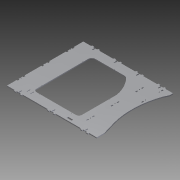
# Autodesk Inventor part: lateral esquerra
Saved by Autodesk Inventor 2012 SP1 (Build 160190100, 190)
## iProperties
Created: 2014-12-15
Part Number: lateral esquerra
Material: Default
Document SubType Name: Modeling
Designer: PRINCIPAL
Density: 1 g/cm^3
Author: PRINCIPAL
Autodesk Inventor part; units mm, degrees
ref_plane "YZ Plane" through (0, 0, 0) normal (1, 0, 0) x (0, 1, 0)
ref_plane "XZ Plane" through (0, 0, 0) normal (0, 1, 0) x (-1, 0, 0)
sketch "Boceto1" plane through (0, 0, 0) normal (0, 0, 1) x (1, 0, 0)
  line L0 (-98.625, -84.15) -> (-98.625, -94.05)
  line L1 (-98.625, -94.05) -> (-103.575, -94.05)
  line L2 (-103.575, -94.05) -> (-103.575, -84.15)
  line L3 (-103.575, -84.15) -> (-98.625, -84.15)
  line L4 (-98.625, -209.15) -> (-98.625, -219.05)
  line L5 (-98.625, -219.05) -> (-103.575, -219.05)
  line L6 (-103.575, -219.05) -> (-103.575, -209.15)
  line L7 (-103.575, -209.15) -> (-98.625, -209.15)
  line L8 (-98.625, -334.15) -> (-98.625, -344.05)
  line L9 (-98.625, -344.05) -> (-103.575, -344.05)
  line L10 (-103.575, -344.05) -> (-103.575, -334.15)
  line L11 (-103.575, -334.15) -> (-98.625, -334.15)
  line L12 (-98.625, -304.15) -> (-98.625, -314.05)
  line L13 (-98.625, -314.05) -> (-103.575, -314.05)
  line L14 (-103.575, -314.05) -> (-103.575, -304.15)
  line L15 (-103.575, -304.15) -> (-98.625, -304.15)
  line L16 (-98.625, -179.15) -> (-98.625, -189.05)
  line L17 (-98.625, -189.05) -> (-103.575, -189.05)
  line L18 (-103.575, -189.05) -> (-103.575, -179.15)
  line L19 (-103.575, -179.15) -> (-98.625, -179.15)
  line L20 (-98.625, -54.15) -> (-98.625, -64.05)
  line L21 (-98.625, -64.05) -> (-103.575, -64.05)
  line L22 (-103.575, -64.05) -> (-103.575, -54.15)
  line L23 (-103.575, -54.15) -> (-98.625, -54.15)
  arc A0 (-453.6069, -72.1) -> (-455.6069, -74.1) centre (-453.6069, -74.1) ccw
  arc A1 (-455.6069, -74.1) -> (-453.6069, -76.1) centre (-453.6069, -74.1) ccw
  arc A2 (-453.6069, -76.1) -> (-451.6069, -74.1) centre (-453.6069, -74.1) ccw
  arc A3 (-451.6069, -74.1) -> (-453.6069, -72.1) centre (-453.6069, -74.1) ccw
  arc A4 (-453.6069, -322.0506) -> (-455.6069, -324.0506) centre (-453.6069, -324.0506) ccw
  arc A5 (-455.6069, -324.0506) -> (-451.6069, -324.0506) centre (-453.6069, -324.051) ccw
  arc A6 (-451.6069, -324.0506) -> (-451.6069, -324.0506) centre (-453.6069, -324.0506) ccw
  arc A7 (-451.6069, -324.0506) -> (-453.6069, -322.0506) centre (-453.6069, -324.0506) ccw
  arc A8 (-453.6069, -197.1) -> (-455.6069, -199.1) centre (-453.6069, -199.1) ccw
  arc A9 (-455.6069, -199.1) -> (-453.6069, -201.1) centre (-453.6069, -199.1) ccw
  arc A10 (-453.6069, -201.1) -> (-451.6069, -199.1) centre (-453.6069, -199.1) ccw
  arc A11 (-451.6069, -199.1) -> (-453.6069, -197.1) centre (-453.6069, -199.1) ccw
  arc A12 (-101.1, -197.1) -> (-103.1, -199.1) centre (-101.1, -199.1) ccw
  arc A13 (-103.1, -199.1) -> (-101.1, -201.1) centre (-101.1, -199.1) ccw
  arc A14 (-101.1, -201.1) -> (-99.1, -199.1) centre (-101.1, -199.1) ccw
  arc A15 (-99.1, -199.1) -> (-101.1, -197.1) centre (-101.1, -199.1) ccw
  arc A16 (-101.1, -322.1) -> (-103.1, -324.1) centre (-101.1, -324.1) ccw
  arc A17 (-103.1, -324.1) -> (-101.1, -326.1) centre (-101.1, -324.1) ccw
  arc A18 (-101.1, -326.1) -> (-99.1, -324.1) centre (-101.1, -324.1) ccw
  arc A19 (-99.1, -324.1) -> (-101.1, -322.1) centre (-101.1, -324.1) ccw
  arc A20 (-101.1, -72.1) -> (-103.1, -74.1) centre (-101.1, -74.1) ccw
  arc A21 (-103.1, -74.1) -> (-101.1, -76.1) centre (-101.1, -74.1) ccw
  arc A22 (-101.1, -76.1) -> (-99.1, -74.1) centre (-101.1, -74.1) ccw
  arc A23 (-99.1, -74.1) -> (-101.1, -72.1) centre (-101.1, -74.1) ccw
  line L24 (-380.769, -353.9818) -> (-380.769, -368.4554)
  line L25 (-380.769, -368.4554) -> (-380.7613, -368.586)
  line L26 (-380.7613, -368.586) -> (-380.7385, -368.7128)
  line L27 (-380.7385, -368.7128) -> (-380.7016, -368.8352)
  line L28 (-380.7016, -368.8352) -> (-380.6511, -368.9525)
  line L29 (-380.6511, -368.9525) -> (-380.588, -369.0641)
  line L30 (-380.588, -369.0641) -> (-380.5128, -369.1694)
  line L31 (-380.5128, -369.1694) -> (-380.4265, -369.2678)
  line L32 (-380.4265, -369.2678) -> (-380.3297, -369.3584)
  line L33 (-380.3297, -369.3584) -> (-380.2231, -369.4409)
  line L34 (-380.2231, -369.4409) -> (-380.1077, -369.5144)
  line L35 (-380.1077, -369.5144) -> (-379.984, -369.5784)
  line L36 (-379.984, -369.5784) -> (-379.8529, -369.6321)
  line L37 (-379.8529, -369.6321) -> (-379.7151, -369.6751)
  line L38 (-379.7151, -369.6751) -> (-379.5713, -369.7065)
  line L39 (-379.5713, -369.7065) -> (-379.4224, -369.7259)
  line L40 (-379.4224, -369.7259) -> (-379.269, -369.7325)
  line L41 (-379.269, -369.7325) -> (-379.169, -369.7325)
  line L42 (-379.169, -369.7325) -> (-379.0156, -369.7259)
  line L43 (-379.0156, -369.7259) -> (-378.8667, -369.7065)
  line L44 (-378.8667, -369.7065) -> (-378.723, -369.6751)
  line L45 (-378.723, -369.6751) -> (-378.5851, -369.6321)
  line L46 (-378.5851, -369.6321) -> (-378.454, -369.5784)
  line L47 (-378.454, -369.5784) -> (-378.3303, -369.5144)
  line L48 (-378.3303, -369.5144) -> (-378.2149, -369.4409)
  line L49 (-378.2149, -369.4409) -> (-378.1083, -369.3584)
  line L50 (-378.1083, -369.3584) -> (-378.0115, -369.2678)
  line L51 (-378.0115, -369.2678) -> (-377.9252, -369.1694)
  line L52 (-377.9252, -369.1694) -> (-377.85, -369.0641)
  line L53 (-377.85, -369.0641) -> (-377.7869, -368.9525)
  line L54 (-377.7869, -368.9525) -> (-377.7364, -368.8352)
  line L55 (-377.7364, -368.8352) -> (-377.6995, -368.7128)
  line L56 (-377.6995, -368.7128) -> (-377.6768, -368.586)
  line L57 (-377.6768, -368.586) -> (-377.669, -368.4554)
  line L58 (-377.669, -368.4554) -> (-377.669, -353.9818)
  line L59 (-377.669, -353.9818) -> (-377.6768, -353.8512)
  line L60 (-377.6768, -353.8512) -> (-377.6995, -353.7244)
  line L61 (-377.6995, -353.7244) -> (-377.7364, -353.602)
  line L62 (-377.7364, -353.602) -> (-377.7869, -353.4847)
  line L63 (-377.7869, -353.4847) -> (-377.85, -353.373)
  line L64 (-377.85, -353.373) -> (-377.9252, -353.2677)
  line L65 (-377.9252, -353.2677) -> (-378.0115, -353.1694)
  line L66 (-378.0115, -353.1694) -> (-378.1083, -353.0787)
  line L67 (-378.1083, -353.0787) -> (-378.2149, -352.9963)
  line L68 (-378.2149, -352.9963) -> (-378.3303, -352.9228)
  line L69 (-378.3303, -352.9228) -> (-378.454, -352.8588)
  line L70 (-378.454, -352.8588) -> (-378.5851, -352.805)
  line L71 (-378.5851, -352.805) -> (-378.723, -352.7621)
  line L72 (-378.723, -352.7621) -> (-378.8667, -352.7306)
  line L73 (-378.8667, -352.7306) -> (-379.0156, -352.7113)
  line L74 (-379.0156, -352.7113) -> (-379.169, -352.7047)
  line L75 (-379.169, -352.7047) -> (-379.269, -352.7047)
  line L76 (-379.269, -352.7047) -> (-379.4224, -352.7113)
  line L77 (-379.4224, -352.7113) -> (-379.5713, -352.7306)
  line L78 (-379.5713, -352.7306) -> (-379.7151, -352.7621)
  line L79 (-379.7151, -352.7621) -> (-379.8529, -352.805)
  line L80 (-379.8529, -352.805) -> (-379.984, -352.8588)
  line L81 (-379.984, -352.8588) -> (-380.1077, -352.9228)
  line L82 (-380.1077, -352.9228) -> (-380.2231, -352.9963)
  line L83 (-380.2231, -352.9963) -> (-380.3297, -353.0787)
  line L84 (-380.3297, -353.0787) -> (-380.4265, -353.1694)
  line L85 (-380.4265, -353.1694) -> (-380.5128, -353.2677)
  line L86 (-380.5128, -353.2677) -> (-380.588, -353.373)
  line L87 (-380.588, -353.373) -> (-380.6511, -353.4847)
  line L88 (-380.6511, -353.4847) -> (-380.7016, -353.602)
  line L89 (-380.7016, -353.602) -> (-380.7385, -353.7244)
  line L90 (-380.7385, -353.7244) -> (-380.7613, -353.8512)
  line L91 (-380.7613, -353.8512) -> (-380.769, -353.9818)
  line L92 (-151.6064, -347.1) -> (-352.0892, -347.1)
  arc A24 (-367.0892, -332.1) -> (-352.0892, -347.1) centre (-352.0892, -332.1) ccw
  line L93 (-367.0892, -332.1) -> (-367.0892, -71.1)
  arc A25 (-347.0892, -51.1) -> (-367.0892, -71.1) centre (-347.0892, -71.1) ccw
  line L94 (-347.0892, -51.1) -> (-200.6138, -51.1)
  arc A26 (-186.1017, -57.3377) -> (-200.6138, -51.1) centre (-200.6138, -71.1) ccw
  arc A27 (-136.6064, -154.1) -> (-186.1017, -57.3377) centre (-325.8382, -189.8548) ccw
  line L95 (-136.6064, -154.1) -> (-136.6064, -332.1)
  arc A28 (-151.6064, -347.1) -> (-136.6064, -332.1) centre (-151.6064, -332.1) ccw
  line L96 (-361.769, -353.9818) -> (-361.769, -368.4554)
  line L97 (-361.769, -368.4554) -> (-361.7613, -368.586)
  line L98 (-361.7613, -368.586) -> (-361.7385, -368.7128)
  line L99 (-361.7385, -368.7128) -> (-361.7016, -368.8352)
  line L100 (-361.7016, -368.8352) -> (-361.6511, -368.9525)
  line L101 (-361.6511, -368.9525) -> (-361.588, -369.0641)
  line L102 (-361.588, -369.0641) -> (-361.5128, -369.1694)
  line L103 (-361.5128, -369.1694) -> (-361.4265, -369.2678)
  line L104 (-361.4265, -369.2678) -> (-361.3297, -369.3584)
  line L105 (-361.3297, -369.3584) -> (-361.2231, -369.4409)
  line L106 (-361.2231, -369.4409) -> (-361.1077, -369.5144)
  line L107 (-361.1077, -369.5144) -> (-360.984, -369.5784)
  line L108 (-360.984, -369.5784) -> (-360.8529, -369.6321)
  line L109 (-360.8529, -369.6321) -> (-360.7151, -369.6751)
  line L110 (-360.7151, -369.6751) -> (-360.5713, -369.7065)
  line L111 (-360.5713, -369.7065) -> (-360.4224, -369.7259)
  line L112 (-360.4224, -369.7259) -> (-360.269, -369.7325)
  line L113 (-360.269, -369.7325) -> (-360.169, -369.7325)
  line L114 (-360.169, -369.7325) -> (-360.0156, -369.7259)
  line L115 (-360.0156, -369.7259) -> (-359.8667, -369.7065)
  line L116 (-359.8667, -369.7065) -> (-359.723, -369.6751)
  line L117 (-359.723, -369.6751) -> (-359.5851, -369.6321)
  line L118 (-359.5851, -369.6321) -> (-359.454, -369.5784)
  line L119 (-359.454, -369.5784) -> (-359.3303, -369.5144)
  line L120 (-359.3303, -369.5144) -> (-359.2149, -369.4409)
  line L121 (-359.2149, -369.4409) -> (-359.1083, -369.3584)
  line L122 (-359.1083, -369.3584) -> (-359.0115, -369.2678)
  line L123 (-359.0115, -369.2678) -> (-358.9252, -369.1694)
  line L124 (-358.9252, -369.1694) -> (-358.85, -369.0641)
  line L125 (-358.85, -369.0641) -> (-358.7869, -368.9525)
  line L126 (-358.7869, -368.9525) -> (-358.7364, -368.8352)
  line L127 (-358.7364, -368.8352) -> (-358.6995, -368.7128)
  line L128 (-358.6995, -368.7128) -> (-358.6768, -368.586)
  line L129 (-358.6768, -368.586) -> (-358.669, -368.4554)
  line L130 (-358.669, -368.4554) -> (-358.669, -353.9818)
  line L131 (-358.669, -353.9818) -> (-358.6768, -353.8512)
  line L132 (-358.6768, -353.8512) -> (-358.6995, -353.7244)
  line L133 (-358.6995, -353.7244) -> (-358.7364, -353.602)
  line L134 (-358.7364, -353.602) -> (-358.7869, -353.4847)
  line L135 (-358.7869, -353.4847) -> (-358.85, -353.373)
  line L136 (-358.85, -353.373) -> (-358.9252, -353.2677)
  line L137 (-358.9252, -353.2677) -> (-359.0115, -353.1694)
  line L138 (-359.0115, -353.1694) -> (-359.1083, -353.0787)
  line L139 (-359.1083, -353.0787) -> (-359.2149, -352.9963)
  line L140 (-359.2149, -352.9963) -> (-359.3303, -352.9228)
  line L141 (-359.3303, -352.9228) -> (-359.454, -352.8588)
  line L142 (-359.454, -352.8588) -> (-359.5851, -352.805)
  line L143 (-359.5851, -352.805) -> (-359.723, -352.7621)
  line L144 (-359.723, -352.7621) -> (-359.8667, -352.7306)
  line L145 (-359.8667, -352.7306) -> (-360.0156, -352.7113)
  line L146 (-360.0156, -352.7113) -> (-360.169, -352.7047)
  line L147 (-360.169, -352.7047) -> (-360.269, -352.7047)
  line L148 (-360.269, -352.7047) -> (-360.4224, -352.7113)
  line L149 (-360.4224, -352.7113) -> (-360.5713, -352.7306)
  line L150 (-360.5713, -352.7306) -> (-360.7151, -352.7621)
  line L151 (-360.7151, -352.7621) -> (-360.8529, -352.805)
  line L152 (-360.8529, -352.805) -> (-360.984, -352.8588)
  line L153 (-360.984, -352.8588) -> (-361.1077, -352.9228)
  line L154 (-361.1077, -352.9228) -> (-361.2231, -352.9963)
  line L155 (-361.2231, -352.9963) -> (-361.3297, -353.0787)
  line L156 (-361.3297, -353.0787) -> (-361.4265, -353.1694)
  line L157 (-361.4265, -353.1694) -> (-361.5128, -353.2677)
  line L158 (-361.5128, -353.2677) -> (-361.588, -353.373)
  line L159 (-361.588, -353.373) -> (-361.6511, -353.4847)
  line L160 (-361.6511, -353.4847) -> (-361.7016, -353.602)
  line L161 (-361.7016, -353.602) -> (-361.7385, -353.7244)
  line L162 (-361.7385, -353.7244) -> (-361.7613, -353.8512)
  line L163 (-361.7613, -353.8512) -> (-361.769, -353.9818)
  line L164 (-172.1123, -393.2) -> (-80.2, -393.2)
  line L165 (-80.2, -393.2) -> (-80.2, -398.2)
  line L166 (-80.2, -398.2) -> (-69.9334, -398.2)
  line L167 (-69.9334, -398.2) -> (-69.9334, -393.2)
  line L168 (-69.9334, -393.2) -> (-62.1933, -393.2)
  line L169 (-62.1933, -393.2) -> (-62.1933, -387)
  line L170 (-62.1933, -387) -> (-63.4433, -387)
  line L171 (-63.4433, -387) -> (-63.4433, -384)
  line L172 (-63.4433, -384) -> (-62.1933, -384)
  line L173 (-62.1933, -384) -> (-62.1933, -378.3312)
  line L174 (-62.1933, -378.3312) -> (-58.1, -378.3312)
  line L175 (-58.1, -378.3312) -> (-58.1, -384)
  line L176 (-58.1, -384) -> (-56.85, -384)
  line L177 (-56.85, -384) -> (-56.85, -387)
  line L178 (-56.85, -387) -> (-58.1, -387)
  line L179 (-58.1, -387) -> (-58.1, -393.2)
  line L180 (-58.1, -393.2) -> (-50.2, -393.2)
  line L181 (-50.2, -393.2) -> (-50.2, -398.2)
  line L182 (-50.2, -398.2) -> (-39.9334, -398.2)
  line L183 (-39.9334, -398.2) -> (-39.9334, -393.2)
  line L184 (-39.9334, -393.2) -> (0, -393.2)
  line L185 (0, -393.2) -> (0, -352.5849)
  arc A29 (-10.9058, -314.7908) -> (0, -352.5849) centre (1010.3894, -40.5586) ccw
  arc A30 (-10.9058, -45.4092) -> (-10.9058, -314.7908) centre (375.2905, -180.1) ccw
  arc A31 (0, -22.2232) -> (-10.9058, -45.4092) centre (46137.4522, -21737.6131) ccw
  line L186 (0, -22.2232) -> (0, -5)
  line L187 (0, -5) -> (-40, -5)
  line L188 (-40, -5) -> (-40, 0)
  line L189 (-40, 0) -> (-50.2666, 0)
  line L190 (-50.2666, 0) -> (-50.2666, -5)
  line L191 (-50.2666, -5) -> (-58.1, -5)
  line L192 (-58.1, -5) -> (-58.1, -11.2)
  line L193 (-58.1, -11.2) -> (-56.85, -11.2)
  line L194 (-56.85, -11.2) -> (-56.85, -14.2)
  line L195 (-56.85, -14.2) -> (-58.1, -14.2)
  line L196 (-58.1, -14.2) -> (-58.1, -19.8688)
  line L197 (-58.1, -19.8688) -> (-62.1933, -19.8688)
  line L198 (-62.1933, -19.8688) -> (-62.1933, -14.2)
  line L199 (-62.1933, -14.2) -> (-63.4433, -14.2)
  line L200 (-63.4433, -14.2) -> (-63.4433, -11.2)
  line L201 (-63.4433, -11.2) -> (-62.1933, -11.2)
  line L202 (-62.1933, -11.2) -> (-62.1933, -5)
  line L203 (-62.1933, -5) -> (-70, -5)
  line L204 (-70, -5) -> (-70, 0)
  line L205 (-70, 0) -> (-80.2666, 0)
  line L206 (-80.2666, 0) -> (-80.2666, -5)
  line L207 (-80.2666, -5) -> (-152, -5)
  line L208 (-152, -5) -> (-152, 0)
  line L209 (-152, 0) -> (-162.2666, 0)
  line L210 (-162.2666, 0) -> (-162.2666, -5)
  line L211 (-162.2666, -5) -> (-170.1, -5)
  line L212 (-170.1, -5) -> (-170.1, -11.2)
  line L213 (-170.1, -11.2) -> (-168.85, -11.2)
  line L214 (-168.85, -11.2) -> (-168.85, -14.2)
  line L215 (-168.85, -14.2) -> (-170.1, -14.2)
  line L216 (-170.1, -14.2) -> (-170.1, -19.8688)
  line L217 (-170.1, -19.8688) -> (-174.1933, -19.8688)
  line L218 (-174.1933, -19.8688) -> (-174.1933, -14.2)
  line L219 (-174.1933, -14.2) -> (-175.4433, -14.2)
  line L220 (-175.4433, -14.2) -> (-175.4433, -11.2)
  line L221 (-175.4433, -11.2) -> (-174.1933, -11.2)
  line L222 (-174.1933, -11.2) -> (-174.1933, -5)
  line L223 (-174.1933, -5) -> (-182, -5)
  line L224 (-182, -5) -> (-182, 0)
  line L225 (-182, 0) -> (-192.2666, 0)
  line L226 (-192.2666, 0) -> (-192.2666, -5)
  line L227 (-192.2666, -5) -> (-264, -5)
  line L228 (-264, -5) -> (-264, 0)
  line L229 (-264, 0) -> (-274.2666, 0)
  line L230 (-274.2666, 0) -> (-274.2666, -5)
  line L231 (-274.2666, -5) -> (-282.1, -5)
  line L232 (-282.1, -5) -> (-282.1, -11.2)
  line L233 (-282.1, -11.2) -> (-280.85, -11.2)
  line L234 (-280.85, -11.2) -> (-280.85, -14.2)
  line L235 (-280.85, -14.2) -> (-282.1, -14.2)
  line L236 (-282.1, -14.2) -> (-282.1, -19.8688)
  line L237 (-282.1, -19.8688) -> (-286.1933, -19.8688)
  line L238 (-286.1933, -19.8688) -> (-286.1933, -14.2)
  line L239 (-286.1933, -14.2) -> (-287.4433, -14.2)
  line L240 (-287.4433, -14.2) -> (-287.4433, -11.2)
  line L241 (-287.4433, -11.2) -> (-286.1933, -11.2)
  line L242 (-286.1933, -11.2) -> (-286.1933, -5)
  line L243 (-286.1933, -5) -> (-294, -5)
  line L244 (-294, -5) -> (-294, 0)
  line L245 (-294, 0) -> (-304.2666, 0)
  line L246 (-304.2666, 0) -> (-304.2666, -5)
  line L247 (-304.2666, -5) -> (-376, -5)
  line L248 (-376, -5) -> (-376, 0)
  line L249 (-376, 0) -> (-386.2666, 0)
  line L250 (-386.2666, 0) -> (-386.2666, -5)
  line L251 (-386.2666, -5) -> (-394.1, -5)
  line L252 (-394.1, -5) -> (-394.1, -11.2)
  line L253 (-394.1, -11.2) -> (-392.85, -11.2)
  line L254 (-392.85, -11.2) -> (-392.85, -14.2)
  line L255 (-392.85, -14.2) -> (-394.1, -14.2)
  line L256 (-394.1, -14.2) -> (-394.1, -19.8688)
  line L257 (-394.1, -19.8688) -> (-398.1933, -19.8688)
  line L258 (-398.1933, -19.8688) -> (-398.1933, -14.2)
  line L259 (-398.1933, -14.2) -> (-399.4433, -14.2)
  line L260 (-399.4433, -14.2) -> (-399.4433, -11.2)
  line L261 (-399.4433, -11.2) -> (-398.1933, -11.2)
  line L262 (-398.1933, -11.2) -> (-398.1933, -5)
  line L263 (-398.1933, -5) -> (-406, -5)
  line L264 (-406, -5) -> (-406, 0)
  line L265 (-406, 0) -> (-416.2666, 0)
  line L266 (-416.2666, 0) -> (-416.2666, -5)
  line L267 (-416.2666, -5) -> (-456.2, -5)
  line L268 (-456.2, -5) -> (-456.2, -54.2)
  line L269 (-456.2, -54.2) -> (-451.2069, -54.2)
  line L270 (-451.2069, -54.2) -> (-451.2069, -64)
  line L271 (-451.2069, -64) -> (-456.2, -64)
  line L272 (-456.2, -64) -> (-456.2, -84.2)
  line L273 (-456.2, -84.2) -> (-451.2069, -84.2)
  line L274 (-451.2069, -84.2) -> (-451.2069, -94)
  line L275 (-451.2069, -94) -> (-456.2069, -94)
  line L276 (-456.2069, -94) -> (-456.2069, -179.2)
  line L277 (-456.2069, -179.2) -> (-451.2069, -179.2)
  line L278 (-451.2069, -179.2) -> (-451.2069, -189)
  line L279 (-451.2069, -189) -> (-456.2069, -189)
  line L280 (-456.2069, -189) -> (-456.2069, -209.2)
  line L281 (-456.2069, -209.2) -> (-451.2069, -209.2)
  line L282 (-451.2069, -209.2) -> (-451.2069, -219)
  line L283 (-451.2069, -219) -> (-456.2069, -219)
  line L284 (-456.2069, -219) -> (-456.2069, -304.2)
  line L285 (-456.2069, -304.2) -> (-451.2069, -304.2)
  line L286 (-451.2069, -304.2) -> (-451.2069, -314)
  line L287 (-451.2069, -314) -> (-456.2069, -314)
  line L288 (-456.2069, -314) -> (-456.2069, -334.2)
  line L289 (-456.2069, -334.2) -> (-451.2069, -334.2)
  line L290 (-451.2069, -334.2) -> (-451.2069, -344)
  line L291 (-451.2069, -344) -> (-456.2, -344)
  line L292 (-456.2, -344) -> (-456.2, -393.2)
  line L293 (-456.2, -393.2) -> (-416.2, -393.2)
  line L294 (-416.2, -393.2) -> (-416.2, -398.2)
  line L295 (-416.2, -398.2) -> (-405.9334, -398.2)
  line L296 (-405.9334, -398.2) -> (-405.9334, -393.2)
  line L297 (-405.9334, -393.2) -> (-398.1933, -393.2)
  line L298 (-398.1933, -393.2) -> (-398.1933, -387)
  line L299 (-398.1933, -387) -> (-399.4433, -387)
  line L300 (-399.4433, -387) -> (-399.4433, -384)
  line L301 (-399.4433, -384) -> (-398.1933, -384)
  line L302 (-398.1933, -384) -> (-398.1933, -378.3312)
  line L303 (-398.1933, -378.3312) -> (-394.1, -378.3312)
  line L304 (-394.1, -378.3312) -> (-394.1, -384)
  line L305 (-394.1, -384) -> (-392.85, -384)
  line L306 (-392.85, -384) -> (-392.85, -387)
  line L307 (-392.85, -387) -> (-394.1, -387)
  line L308 (-394.1, -387) -> (-394.1, -393.2)
  line L309 (-394.1, -393.2) -> (-386.2, -393.2)
  line L310 (-386.2, -393.2) -> (-386.2, -398.2)
  line L311 (-386.2, -398.2) -> (-375.9334, -398.2)
  line L312 (-375.9334, -398.2) -> (-375.9334, -393.2)
  line L313 (-375.9334, -393.2) -> (-346.9956, -393.2)
  line L314 (-346.9956, -393.2) -> (-248.2565, -393.2)
  line L315 (-248.2565, -393.2) -> (-248.2565, -398.2)
  line L316 (-248.2565, -398.2) -> (-238.0038, -398.2)
  line L317 (-238.0038, -398.2) -> (-238.0038, -393.2)
  line L318 (-238.0038, -393.2) -> (-230.1248, -393.2)
  line L319 (-230.1248, -393.2) -> (-230.1248, -386)
  line L320 (-230.1248, -386) -> (-231.3718, -386)
  line L321 (-231.3718, -386) -> (-231.3718, -383)
  line L322 (-231.3718, -383) -> (-230.1248, -383)
  line L323 (-230.1248, -383) -> (-230.1248, -377.3312)
  line L324 (-230.1248, -377.3312) -> (-226.0752, -377.3312)
  line L325 (-226.0752, -377.3312) -> (-226.0752, -383)
  line L326 (-226.0752, -383) -> (-224.8282, -383)
  line L327 (-224.8282, -383) -> (-224.8282, -386)
  line L328 (-224.8282, -386) -> (-226.0752, -386)
  line L329 (-226.0752, -386) -> (-226.0752, -393.2)
  line L330 (-226.0752, -393.2) -> (-218.2197, -393.2)
  line L331 (-218.2197, -393.2) -> (-218.2197, -398.2)
  line L332 (-218.2197, -398.2) -> (-207.9729, -398.2)
  line L333 (-207.9729, -398.2) -> (-207.9729, -393.2)
  line L334 (-207.9729, -393.2) -> (-172.1123, -393.2)
  line L335 (-163.357, -375.5981) -> (-163.357, -383.6019)
  line L336 (-163.357, -383.6019) -> (-137.3531, -383.6019)
  line L337 (-137.3531, -383.6019) -> (-137.3531, -375.5981)
  line L338 (-137.3531, -375.5981) -> (-163.357, -375.5981)
  point P0 (0, 0)
  constraints: 678 end point, 64 point on circle, 32 centre point
ref_plane "Plano de trabajo4" through (0, 0, 5) normal (0, 0, 1) x (1, 0, 0)
sketch "Boceto2" plane through (0, 0, 5) normal (0, 0, 1) x (1, 0, 0)
  line L0 (0, -5) -> (0, -22.2232) projected
  line L1 (-40, -5) -> (0, -5) projected
  circle A0 centre (-40, -35) radius 2.25
  circle A1 centre (-40, -105) radius 2.25
  line L2 (-42.5, -15) -> (-37.5, -15)
  line L3 (-37.5, -15) -> (-37.5, -25)
  line L4 (-37.5, -25) -> (-42.5, -25)
  line L5 (-42.5, -25) -> (-42.5, -15)
  line L6 (-37.5, -115) -> (-42.5, -115)
  line L7 (-42.5, -115) -> (-42.5, -125)
  line L8 (-42.5, -125) -> (-37.5, -125)
  line L9 (-37.5, -125) -> (-37.5, -115)
  point P0 (0, 0)
  dimension "d3" = 4.5
  dimension "d4" = 40
  dimension "d5" = 40
  dimension "d6" = 30
  dimension "d7" = 70
  dimension "d8" = 5
  dimension "d9" = 10
  dimension "d10" = 5
  dimension "d11" = 10
  dimension "d12" = 37.5
  dimension "d13" = 37.5
  dimension "d14" = 10
  dimension "d15" = 10
  constraints: 16 end point, 4 parallel, 2 centre point, 2 horizontal, 2 perpendicular
  measures "d3" diameter of A0
  measures "d4" distance from line of A0.centre L0
  measures "d5" distance from line of L0 A1.centre
  measures "d6" distance from line of A0.centre L1
  measures "d7" distance of A1.centre A0.centre
  measures "d8" distance between parallel lines of L9 L7
  measures "d9" distance between parallel lines of L8 L6
  measures "d10" distance between parallel lines of L3 L5
  measures "d11" distance between parallel lines of L2 L4
  measures "d12" distance from line of L0.end L3
  measures "d13" distance between parallel lines of L0 L9
  measures "d14" distance from line of L6 A1.centre
  measures "d15" distance from line of A0.centre L4
extrude "Extrusión3" add sketch "Boceto1" along normal blind 5
extrude "Extrusión4" cut sketch "Boceto2" against normal blind 5
sketch "Boceto5" plane through (0, 0, 0) normal (0, 0, -1) x (-1, 0, 0)
  line L0 (367.0892, -71.1) -> (367.0892, -332.1) projected
  line L1 (207.9729, -393.2) -> (80.2, -393.2) projected
  line L2 (375.9334, -393.2) -> (248.2565, -393.2) projected
  line L3 (456.2, -344) -> (456.2, -393.2) projected
  line L4 (456.2069, -219) -> (456.2069, -304.2) projected
  line L5 (456.2069, -94) -> (456.2069, -179.2) projected
  line L6 (192.2666, -5) -> (264, -5) projected
  circle A0 centre (333.2, -351.2) radius 1.25
  circle A1 centre (171.2, -351.2) radius 1.25
  circle A2 centre (134.2069, -193.2) radius 1.25
  circle A3 centre (370.2069, -304.2) radius 1.25
  circle A4 centre (251.8392, -49) radius 1.25
  circle A5 centre (370.2069, -96.2) radius 1.25
  point P0 (0, 0)
  dimension "d31" = 42
  dimension "d32" = 42
  dimension "d33" = 162
  dimension "d34" = 123
  dimension "d35" = 86
  dimension "d36" = 86
  dimension "d37" = 297
  dimension "d38" = 208
  dimension "d39" = 115.25
  dimension "d40" = 44
  dimension "d41" = 200
  dimension "d42" = 322
  constraints: 6 centre point
  measures "d31" distance from line of A0.centre L2
  measures "d32" distance from line of A1.centre L1
  measures "d33" distance of A0.centre A1.centre
  measures "d34" distance from line of L3 A0.centre
  measures "d35" distance from line of L5 A3.centre
  measures "d36" distance from line of L4 A5.centre
  measures "d37" distance from line of A5.centre L2
  measures "d38" distance of A3.centre A5.centre
  measures "d39" distance from line of A4.centre L0
  measures "d40" distance from line of A4.centre L6
  measures "d41" distance from line of A2.centre L1
  measures "d42" distance from line of L5 A2.centre
extrude "Extrusión5" cut sketch "Boceto5" against normal blind 10
